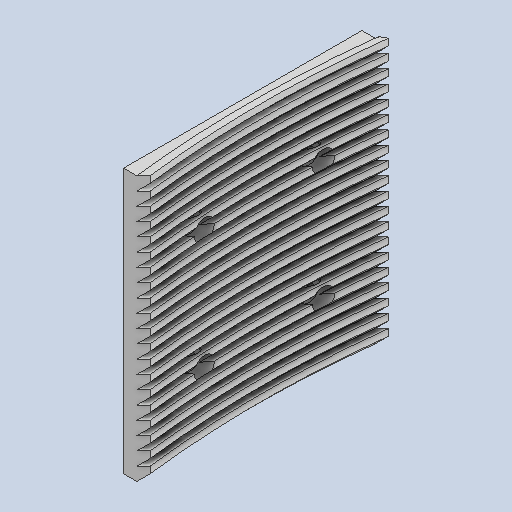
# Autodesk Inventor part: Gripper plate v2
Saved by Autodesk Inventor 2023 (Build 270158000, 158)
## iProperties
Created: 2023-02-14
Part Number: Gripper plate v2
Material: Generic
Document SubType Name: Modeling
Designer: Gabriel - T3 CAD
Density: 1 g/cm^3
Appearance: Default
Author: Gabriel - T3 CAD
Autodesk Inventor part; units mm, degrees
ref_plane "YZ Plane" through (0, 0, 0) normal (1, 0, 0) x (0, 1, 0)
ref_plane "XZ Plane" through (0, 0, 0) normal (0, 1, 0) x (-1, 0, 0)
ref_plane "XY Plane" through (0, 0, 0) normal (0, 0, 1) x (1, 0, 0)
sketch "Sketch1" plane through (0, 0, 0) normal (1, 0, 0) x (0, 1, 0)
  line L0 (0, 0) -> (127, 0)
  line L1 (127, 0) -> (127, 114.3)
  line L2 (127, 114.3) -> (0, 114.3)
  line L3 (0, 114.3) -> (0, 0)
  dimension "d0" = 127
  dimension "d1" = 114.3
  constraints: 8 end point, 2 parallel, 1 horizontal, 1 perpendicular
  measures "d0" distance of L2.end L1.end
  measures "d1" distance of L1.end L0.end
extrude "Extrusion1" add sketch "Sketch1" along normal blind 12.7
sketch "m" plane through (0, 0, 114.3) normal (0, 0, 1) x (1, 0, 0)
  line L0 (0, 0) -> (6.35, 0)
  line L1 (6.35, 0) -> (6.35, 127)
  line L2 (6.35, 127) -> (0, 127)
  line L3 (0, 127) -> (0, 0)
  line L4 (6.35, 0) -> (12.7, 6.35)
  line L5 (12.7, 127) -> (12.7, 0) projected
  line L6 (6.35, 6.35) -> (12.7, 9.525)
  line L7 (0, 0) -> (12.7, 0) projected
  line L8 (6.35, 12.7) -> (12.7, 15.875)
  line L9 (6.35, 6.35) -> (12.7, 12.7)
  line L10 (6.35, 19.05) -> (12.7, 22.225)
  line L11 (6.35, 12.7) -> (12.7, 19.05)
  line L12 (6.35, 25.4) -> (12.7, 28.575)
  line L13 (6.35, 19.05) -> (12.7, 25.4)
  line L14 (6.35, 31.75) -> (12.7, 34.925)
  line L15 (6.35, 25.4) -> (12.7, 31.75)
  line L16 (6.35, 38.1) -> (12.7, 41.275)
  line L17 (6.35, 31.75) -> (12.7, 38.1)
  line L18 (6.35, 44.45) -> (12.7, 47.625)
  line L19 (6.35, 38.1) -> (12.7, 44.45)
  line L20 (6.35, 50.8) -> (12.7, 53.975)
  line L21 (6.35, 44.45) -> (12.7, 50.8)
  line L22 (6.35, 57.15) -> (12.7, 60.325)
  line L23 (6.35, 50.8) -> (12.7, 57.15)
  line L24 (6.35, 63.5) -> (12.7, 66.675)
  line L25 (6.35, 57.15) -> (12.7, 63.5)
  line L26 (6.35, 69.85) -> (12.7, 73.025)
  line L27 (6.35, 63.5) -> (12.7, 69.85)
  line L28 (6.35, 76.2) -> (12.7, 79.375)
  line L29 (6.35, 69.85) -> (12.7, 76.2)
  line L30 (6.35, 82.55) -> (12.7, 85.725)
  line L31 (6.35, 76.2) -> (12.7, 82.55)
  line L32 (6.35, 88.9) -> (12.7, 92.075)
  line L33 (6.35, 82.55) -> (12.7, 88.9)
  line L34 (6.35, 95.25) -> (12.7, 98.425)
  line L35 (6.35, 88.9) -> (12.7, 95.25)
  line L36 (6.35, 101.6) -> (12.7, 104.775)
  line L37 (6.35, 95.25) -> (12.7, 101.6)
  line L38 (6.35, 107.95) -> (12.7, 111.125)
  line L39 (6.35, 101.6) -> (12.7, 107.95)
  line L40 (6.35, 114.3) -> (12.7, 117.475)
  line L41 (6.35, 107.95) -> (12.7, 114.3)
  line L42 (6.35, 120.65) -> (12.7, 123.825)
  line L43 (6.35, 114.3) -> (12.7, 120.65)
  line L44 (6.35, 127) -> (12.7, 130.175)
  line L45 (6.35, 120.65) -> (12.7, 127)
  line L46 (12.7, 127) -> (12.7, 130.175)
  line L47 (12.7, 130.175) -> (12.7, 0)
  line L48 (12.7, 0) -> (38.1, 0)
  line L49 (38.1, 0) -> (38.1, 130.175)
  line L50 (38.1, 130.175) -> (12.7, 130.175)
  dimension "d4" = 6.35
  dimension "d5" = 127
  dimension "d10" = 6.35
  dimension "d11" = 3.175
  dimension "d12" = 45
  dimension "d15" = 6.35
  dimension "d24" = 25.4
  constraints: 98 end point, 76 vertical alignment, 42 parallel, 2 perpendicular, 2 point on line, 1 horizontal, 1 midpoint, 3 other
  measures "d4" distance of L2.end L1.end
  measures "d5" distance of L1.end L0.end
  measures "d10" distance of L6.start point (6.35, 0)
  measures "d11" distance of L6.end L4.end
  measures "d12" angle of L1 L4
  measures "d15" distance of L6.start L8.start
  measures "d24" distance of L48.end L7.end
sketch "Sketch3" plane through (0, 127, 114.3) normal (0, 1, 0) x (1, 0, 0)
  arc A0 (12.7, 114.3) -> (12.7, 0) centre (491.9042, 57.15) ccw
  line L0 (491.9042, 57.15) -> (12.7, 0)
  line L1 (491.9042, 57.15) -> (12.7, 114.3)
  point P0 (0, 0)
  point P1 (0, 114.3)
  constraints: 4 end point, 2 point on circle, 1 centre point
sweep "Sweep1" add profiles "m" path "Sketch3" path curves A0 contours L44 L46 L45 L1
sweep "Sweep2" cut profiles "m" path "Sketch3" path curves A0 contours L4 L5 L7 | L9 L5 L6 | L5 L46 L50 L49 L48 | L11 L5 L8 | L45 L5 L42 | L13 L5 L10 | L43 L5 L40 | L15 L5 L12 | L41 L5 L38 | L17 L5 L14 | L39 L5 L36 | L19 L5 L16 | L37 L5 L34 | L21 L5 L18 | L35 L5 L32 | L23 L5 L20 | L33 L5 L30 | L25 L5 L22 | L31 L5 L28 | L27 L5 L24 | L29 L5 L26
sketch "Sketch4" plane through (0, 0, 0) normal (-1, 0, 0) x (0, 0, 1)
  circle A0 centre (85.725, 34.925) radius 2.5797
  line L0 (114.3, 0) -> (0, 0) projected
  line L1 (0, 0) -> (-18.278, 0)
  line L2 (-18.278, 0) -> (-18.278, 26.1911)
  circle A1 centre (85.725, 92.075) radius 2.5797
  circle A2 centre (28.575, 34.925) radius 2.5797
  circle A3 centre (28.575, 92.075) radius 2.5797
  line L3 (114.3, 127) -> (114.3, 0) projected
  circle A4 centre (85.725, 34.925) radius 5.08
  circle A5 centre (28.575, 34.925) radius 5.08
  circle A6 centre (85.725, 92.075) radius 5.08
  circle A7 centre (28.575, 92.075) radius 5.08
  dimension "d37" = 57.15
  dimension "d40" = 57.15
  dimension "d43" = 28.575
  dimension "d44" = 34.925
  dimension "d45" = 5.1594
  dimension "d46" = 10.16
  dimension "d49" = 57.15
  dimension "d52" = 57.15
  constraints: 8 centre point, 4 end point, 2 horizontal, 2 vertical, 1 coincident, 1 collinear, 1 perpendicular, 12 other
  measures "d37" distance of A0.centre A1.centre
  measures "d40" distance of A0.centre A2.centre
  measures "d43" distance from line of L3 A0.centre
  measures "d44" distance from line of L0 A0.centre
  measures "d45" diameter of A0
  measures "d46" diameter of A4
  measures "d49" distance of A4.centre A5.centre
  measures "d52" distance of A4.centre A6.centre
extrude "Extrusion2" cut sketch "Sketch4" against normal blind 50.8 contours A0 | A1 | A2 | A3 | A4 | A5 | A6 | A7
extrude "Extrusion3" add sketch "Sketch4" against normal blind 3.175
equation "\"d11\" = 0.5 * d10"
body "Solid1"
